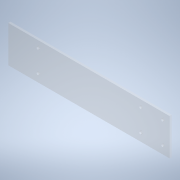
# Autodesk Inventor part: arm1
Saved by Autodesk Inventor 2021 (Build 250183000, 183)
## iProperties
Created: 2022-05-21
Part Number: arm1
Material: Polycarbonate, Clear
Document SubType Name: Modeling
Designer: techv
Mass: 44.8982 g
Surface Area: 268.565 cm^2
Volume: 37.4152 cm^3
Density: 1.2 g/cm^3
Appearance: Polycarbonate - Clear
Author: techv
Autodesk Inventor part; units mm, degrees
ref_plane "YZ Plane" through (0, 0, 0) normal (1, 0, 0) x (0, 1, 0)
ref_plane "XZ Plane" through (0, 0, 0) normal (0, 1, 0) x (-1, 0, 0)
ref_plane "XY Plane" through (0, 0, 0) normal (0, 0, 1) x (1, 0, 0)
sketch "Sketch1" plane through (0, 0, 0) normal (0, 0, 1) x (1, 0, 0)
  circle A0 centre (6.0619, 42.5) radius 1.5 projected
  circle A1 centre (6.0619, 7.5) radius 1.5 projected
  circle A2 centre (28.8092, 42.5) radius 1.5 projected
  circle A3 centre (28.8092, 7.5) radius 1.5 projected
  line L0 (34.8712, 0) -> (0, 0) projected
  line L1 (34.8712, 0) -> (34.8712, 50) projected
  line L2 (0, 50) -> (34.8712, 50) projected
  line L3 (0, 0) -> (0, 50) projected
  line L4 (0, 0) -> (220, 0)
  line L5 (220, 0) -> (220, 50)
  line L6 (220, 50) -> (0, 50)
  line L7 (0, 50) -> (0, 0)
  point P0 (19, 50)
  point P1 (19, 0)
  dimension "d0" = 220
  dimension "d1" = 50
  constraints: 8 end point, 2 parallel, 1 horizontal, 1 perpendicular
  measures "d0" distance of L6.end L5.end
  measures "d1" distance of L5.end L4.end
extrude "Extrusion1" add sketch "Sketch1" along normal blind 3 contours A0 | A1 | A2 | A3 | L0 L3 L2 L1 | L1 L6 L5 L4
sketch "Sketch2" plane through (0, 0, 0) normal (0, 0, -1) x (-1, 0, 0)
  arc A0 (-300, 50) -> (-310, 40) centre (-300, 40) ccw projected
  line L0 (-310, 40) -> (-310, 10) projected
  arc A1 (-310, 10) -> (-300, 0) centre (-300, 10) ccw projected
  line L1 (-300, 0) -> (-170, 0) projected
  line L2 (-170, 0) -> (-170, 50) projected
  line L3 (-170, 50) -> (-300, 50) projected
  circle A2 centre (-250.5156, 19.2053) radius 1.75 projected
  circle A3 centre (-250.7947, 30.5156) radius 1.75 projected
  circle A4 centre (-239.2053, 19.4844) radius 1.75 projected
  circle A5 centre (-239.4844, 30.7947) radius 1.75 projected
  circle A6 centre (-263.75, 25) radius 2.6 projected
  circle A7 centre (-280, 25) radius 5 projected
  circle A8 centre (-296.25, 25) radius 2.6 projected
  circle A9 centre (-245, 25) radius 5.5 projected
  circle A10 centre (-210, 40) radius 1.5 projected
  circle A11 centre (-210, 10) radius 1.5 projected
  circle A12 centre (-180, 40) radius 1.5 projected
  circle A13 centre (-180, 10) radius 1.5 projected
  line L4 (-50, 0) -> (55, 0) projected
  arc A14 (55, 0) -> (65, 10) centre (55, 10) ccw projected
  line L5 (65, 10) -> (65, 40) projected
  arc A15 (65, 40) -> (55, 50) centre (55, 40) ccw projected
  line L6 (55, 50) -> (-50, 50) projected
  line L7 (-50, 50) -> (-50, 0) projected
  circle A16 centre (-40, 40) radius 1.5 projected
  circle A17 centre (-40, 10) radius 1.5 projected
  circle A18 centre (36, 25) radius 5 projected
  circle A19 centre (19.75, 25) radius 2.6 projected
  circle A20 centre (52.25, 25) radius 2.6 projected
  circle A21 centre (-10, 40) radius 1.5 projected
  circle A22 centre (-10, 10) radius 1.5 projected
  point P0 (0, 0)
extrude "Extrusion2" cut sketch "Sketch2" against normal through all contours A10 | A11 | A12 | A13 | A16 | A17
ref_plane "Work Plane1" through (110, 0, 0) normal (1, 0, 0) x (0, 0, -1)
mirror "Mirror1" about plane through (110, 0, 0) normal (1, 0, 0) of "Extrusion2"
body "Solid1"
